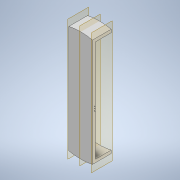
# Autodesk Inventor part: capFor6inchSch40Pipe
Saved by Autodesk Inventor 2021.1 (Build 251245000, 245)
## iProperties
Created: 2020-09-22
Part Number: capFor6inchSch40Pipe
Material: Generic
Document SubType Name: Modeling
Designer: robst
Density: 1 g/cm^3
Appearance: Default
Author: robst
Autodesk Inventor part; units mm, degrees
ref_plane "XZ Plane" through (0, 0, 0) normal (0, 1, 0) x (-1, 0, 0)
ref_plane "XY Plane" through (0, 0, 0) normal (0, 0, 1) x (1, 0, 0)
sketch "Sketch1" plane through (0, 0, 0) normal (0, 0, 1) x (1, 0, 0)
  circle A0 centre (0, 0) radius 84.1375
  circle A1 centre (0, 0) radius 88.9
  dimension "d0" = 168.275
  dimension "d1" = 4.7625
  constraints: 2 centre point, 2 coincident
  measures "d0" diameter of A0
  measures "d1" radial gap between concentric circles of A1 A0
extrude "Extrusion1" add sketch "Sketch1" along normal blind 4.7625 contours A0 | A1
extrude "Extrusion2" add sketch "Sketch1" against normal blind 25.4
sketch "Sketch2" plane through (0, 0, 0) normal (0, 0, -1) x (-1, 0, 0)
  line L0 (-83.5959, 0) -> (84.1375, 0) construction
  circle A0 centre (0, 0) radius 84.1375 construction
  spline S0 degree 2 poles (-77.1102, 1.1002) (-78.0365, 1.1002) (-79.6034, 1.7254) (-80.1746, 2.3506) knots 0 0 0 1 2 2 2
  spline S1 degree 2 poles (-80.1746, 2.3506) (-80.7458, 2.9681) (-81.371, 4.8206) (-81.371, 6.0248) knots 0 0 0 1 2 2 2
  spline S2 degree 2 poles (-81.371, 6.0248) (-81.371, 7.2212) (-80.7612, 8.9965) (-80.1823, 9.6526) knots 0 0 0 1 2 2 2
  spline S3 degree 2 poles (-80.1823, 9.6526) (-79.6111, 10.2933) (-78.0519, 10.9648) (-77.087, 10.9648) knots 0 0 0 1 2 2 2
  spline S4 degree 2 poles (-77.087, 10.9648) (-76.6085, 10.9648) (-75.7671, 10.8259) (-75.4121, 10.7178) knots 0 0 0 1 2 2 2
  spline S5 degree 2 poles (-75.4121, 10.7178) (-75.1033, 10.6175) (-74.4626, 10.3319) (-74.1462, 10.1621) knots 0 0 0 1 2 2 2
  line L1 (-74.1462, 10.1621) -> (-74.1462, 8.6337)
  line L2 (-74.1462, 8.6337) -> (-74.2465, 8.6337)
  spline S6 degree 2 poles (-74.2465, 8.6337) (-74.4163, 8.7881) (-74.9412, 9.2204) (-75.3194, 9.4288) knots 0 0 0 1 2 2 2
  spline S7 degree 2 poles (-75.3194, 9.4288) (-75.6822, 9.6295) (-76.539, 9.8842) (-77.0948, 9.8842) knots 0 0 0 1 2 2 2
  spline S8 degree 2 poles (-77.0948, 9.8842) (-77.7045, 9.8842) (-78.7929, 9.3825) (-79.202, 8.9039) knots 0 0 0 1 2 2 2
  spline S9 degree 2 poles (-79.202, 8.9039) (-79.6034, 8.4176) (-80.0511, 6.9433) (-80.0511, 6.0248) knots 0 0 0 1 2 2 2
  spline S10 degree 2 poles (-80.0511, 6.0248) (-80.0511, 5.0445) (-79.5802, 3.632) (-79.1711, 3.1457) knots 0 0 0 1 2 2 2
  spline S11 degree 2 poles (-79.1711, 3.1457) (-78.7697, 2.6748) (-77.6968, 2.1963) (-77.0948, 2.1963) knots 0 0 0 1 2 2 2
  spline S12 degree 2 poles (-77.0948, 2.1963) (-76.5467, 2.1963) (-75.6127, 2.4664) (-75.25, 2.6671) knots 0 0 0 1 2 2 2
  spline S13 degree 2 poles (-75.25, 2.6671) (-74.9026, 2.8678) (-74.3855, 3.2846) (-74.2388, 3.4313) knots 0 0 0 1 2 2 2
  line L3 (-74.2388, 3.4313) -> (-74.1462, 3.4313)
  line L4 (-74.1462, 3.4313) -> (-74.1462, 1.9184)
  spline S14 degree 2 poles (-74.1462, 1.9184) (-74.4626, 1.7717) (-75.0184, 1.5016) (-75.4121, 1.3781) knots 0 0 0 1 2 2 2
  spline S15 degree 2 poles (-75.4121, 1.3781) (-75.8289, 1.2391) (-76.539, 1.1002) (-77.1102, 1.1002) knots 0 0 0 1 2 2 2
  spline S16 degree 2 poles (-69.0749, 2.0264) (-69.2216, 1.9184) (-69.7156, 1.5324) (-69.9471, 1.4167) knots 0 0 0 1 2 2 2
  spline S17 degree 2 poles (-69.9471, 1.4167) (-70.2636, 1.2468) (-70.858, 1.0693) (-71.3983, 1.0693) knots 0 0 0 1 2 2 2
  spline S18 degree 2 poles (-71.3983, 1.0693) (-71.8383, 1.0693) (-72.6333, 1.4012) (-72.9343, 1.7023) knots 0 0 0 1 2 2 2
  spline S19 degree 2 poles (-72.9343, 1.7023) (-73.2199, 1.9956) (-73.5673, 2.8601) (-73.5673, 3.3386) knots 0 0 0 1 2 2 2
  spline S20 degree 2 poles (-73.5673, 3.3386) (-73.5673, 4.0796) (-72.942, 5.1294) (-72.2628, 5.4304) knots 0 0 0 1 2 2 2
  spline S21 degree 2 poles (-72.2628, 5.4304) (-71.6607, 5.7083) (-70.0243, 5.9167) (-69.0749, 5.9707) knots 0 0 0 1 2 2 2
  line L5 (-69.0749, 5.9707) -> (-69.0749, 6.2023)
  spline S22 degree 2 poles (-69.0749, 6.2023) (-69.0749, 6.6191) (-69.3296, 7.1363) (-69.5612, 7.2829) knots 0 0 0 1 2 2 2
  spline S23 degree 2 poles (-69.5612, 7.2829) (-69.7928, 7.4296) (-70.4566, 7.5222) (-70.8117, 7.5222) knots 0 0 0 1 2 2 2
  spline S24 degree 2 poles (-70.8117, 7.5222) (-71.2285, 7.5222) (-72.3554, 7.2752) (-72.9189, 7.0359) knots 0 0 0 1 2 2 2
  line L6 (-72.9189, 7.0359) -> (-72.9884, 7.0359)
  line L7 (-72.9884, 7.0359) -> (-72.9884, 8.2632)
  spline S25 degree 2 poles (-72.9884, 8.2632) (-72.6564, 8.3559) (-71.4137, 8.5874) (-70.8039, 8.5874) knots 0 0 0 1 2 2 2
  spline S26 degree 2 poles (-70.8039, 8.5874) (-70.0629, 8.5874) (-69.0518, 8.3559) (-68.6504, 8.0548) knots 0 0 0 1 2 2 2
  spline S27 degree 2 poles (-68.6504, 8.0548) (-68.2567, 7.7615) (-67.8708, 6.8275) (-67.8708, 6.156) knots 0 0 0 1 2 2 2
  line L8 (-67.8708, 6.156) -> (-67.8708, 1.27)
  line L9 (-67.8708, 1.27) -> (-69.0749, 1.27)
  line L10 (-69.0749, 1.27) -> (-69.0749, 2.0264)
  line L11 (-69.0749, 3.0299) -> (-69.0749, 5.0136)
  spline S28 degree 2 poles (-69.0749, 5.0136) (-69.5072, 4.975) (-70.8117, 4.8438) (-71.2208, 4.7203) knots 0 0 0 1 2 2 2
  spline S29 degree 2 poles (-71.2208, 4.7203) (-71.6993, 4.5736) (-72.3245, 3.9639) (-72.3245, 3.4235) knots 0 0 0 1 2 2 2
  spline S30 degree 2 poles (-72.3245, 3.4235) (-72.3245, 2.806) (-71.6298, 2.1808) (-70.966, 2.1808) knots 0 0 0 1 2 2 2
  spline S31 degree 2 poles (-70.966, 2.1808) (-70.4026, 2.1808) (-69.4763, 2.6671) (-69.0749, 3.0299) knots 0 0 0 1 2 2 2
  spline S32 degree 2 poles (-60.1906, 5.0368) (-60.1906, 3.246) (-61.8964, 1.1311) (-63.2009, 1.1311) knots 0 0 0 1 2 2 2
  spline S33 degree 2 poles (-63.2009, 1.1311) (-63.7335, 1.1311) (-64.5517, 1.3781) (-64.9762, 1.6328) knots 0 0 0 1 2 2 2
  line L12 (-64.9762, 1.6328) -> (-64.9762, -1.3621)
  line L13 (-64.9762, -1.3621) -> (-66.1804, -1.3621)
  line L14 (-66.1804, -1.3621) -> (-66.1804, 8.4176)
  line L15 (-66.1804, 8.4176) -> (-64.9762, 8.4176)
  line L16 (-64.9762, 8.4176) -> (-64.9762, 7.6689)
  spline S34 degree 2 poles (-64.9762, 7.6689) (-64.5286, 8.078) (-63.4325, 8.6183) (-62.7918, 8.6183) knots 0 0 0 1 2 2 2
  spline S35 degree 2 poles (-62.7918, 8.6183) (-61.5645, 8.6183) (-60.1906, 6.6732) (-60.1906, 5.0368) knots 0 0 0 1 2 2 2
  spline S36 degree 2 poles (-61.4333, 4.8978) (-61.4333, 6.1251) (-62.2129, 7.4759) (-63.0851, 7.4759) knots 0 0 0 1 2 2 2
  spline S37 degree 2 poles (-63.0851, 7.4759) (-63.5946, 7.4759) (-64.5517, 7.0205) (-64.9762, 6.6654) knots 0 0 0 1 2 2 2
  line L17 (-64.9762, 6.6654) -> (-64.9762, 2.6054)
  spline S38 degree 2 poles (-64.9762, 2.6054) (-64.5054, 2.3815) (-63.8339, 2.2117) (-63.4016, 2.2117) knots 0 0 0 1 2 2 2
  spline S39 degree 2 poles (-63.4016, 2.2117) (-62.4676, 2.2117) (-61.4333, 3.5856) (-61.4333, 4.8978) knots 0 0 0 1 2 2 2
  line L18 (-49.0601, 9.6681) -> (-53.4907, 9.6681)
  line L19 (-53.4907, 9.6681) -> (-53.4907, 6.9819)
  line L20 (-53.4907, 6.9819) -> (-49.2453, 6.9819)
  line L21 (-49.2453, 6.9819) -> (-49.2453, 5.855)
  line L22 (-49.2453, 5.855) -> (-53.4907, 5.855)
  line L23 (-53.4907, 5.855) -> (-53.4907, 1.27)
  line L24 (-53.4907, 1.27) -> (-54.7566, 1.27)
  line L25 (-54.7566, 1.27) -> (-54.7566, 10.795)
  line L26 (-54.7566, 10.795) -> (-49.0601, 10.795)
  line L27 (-49.0601, 10.795) -> (-49.0601, 9.6681)
  spline S40 degree 2 poles (-42.144, 4.8438) (-42.144, 3.0376) (-43.8808, 1.0693) (-45.3319, 1.0693) knots 0 0 0 1 2 2 2
  spline S41 degree 2 poles (-45.3319, 1.0693) (-46.8216, 1.0693) (-48.5275, 3.0994) (-48.5275, 4.8438) knots 0 0 0 1 2 2 2
  spline S42 degree 2 poles (-48.5275, 4.8438) (-48.5275, 6.6346) (-46.7676, 8.6183) (-45.3319, 8.6183) knots 0 0 0 1 2 2 2
  spline S43 degree 2 poles (-45.3319, 8.6183) (-43.8808, 8.6183) (-42.144, 6.6423) (-42.144, 4.8438) knots 0 0 0 1 2 2 2
  spline S44 degree 2 poles (-43.3868, 4.8438) (-43.3868, 6.2332) (-44.3979, 7.584) (-45.3319, 7.584) knots 0 0 0 1 2 2 2
  spline S45 degree 2 poles (-45.3319, 7.584) (-46.2659, 7.584) (-47.2848, 6.2332) (-47.2848, 4.8438) knots 0 0 0 1 2 2 2
  spline S46 degree 2 poles (-47.2848, 4.8438) (-47.2848, 3.493) (-46.2659, 2.1036) (-45.3319, 2.1036) knots 0 0 0 1 2 2 2
  spline S47 degree 2 poles (-45.3319, 2.1036) (-44.4056, 2.1036) (-43.3868, 3.4699) (-43.3868, 4.8438) knots 0 0 0 1 2 2 2
  line L28 (-37.1191, 7.1286) -> (-37.1808, 7.1286)
  spline S48 degree 2 poles (-37.1808, 7.1286) (-37.3198, 7.1672) (-37.6208, 7.1826) (-37.8292, 7.1826) knots 0 0 0 1 2 2 2
  spline S49 degree 2 poles (-37.8292, 7.1826) (-38.3155, 7.1826) (-39.2726, 6.7581) (-39.7049, 6.3413) knots 0 0 0 1 2 2 2
  line L29 (-39.7049, 6.3413) -> (-39.7049, 1.27)
  line L30 (-39.7049, 1.27) -> (-40.909, 1.27)
  line L31 (-40.909, 1.27) -> (-40.909, 8.4176)
  line L32 (-40.909, 8.4176) -> (-39.7049, 8.4176)
  line L33 (-39.7049, 8.4176) -> (-39.7049, 7.3524)
  spline S50 degree 2 poles (-39.7049, 7.3524) (-39.0488, 7.939) (-38.0685, 8.4176) (-37.6054, 8.4176) knots 0 0 0 1 2 2 2
  spline S51 degree 2 poles (-37.6054, 8.4176) (-37.4201, 8.4176) (-37.2349, 8.4022) (-37.1191, 8.379) knots 0 0 0 1 2 2 2
  line L34 (-37.1191, 8.379) -> (-37.1191, 7.1286)
  spline S52 degree 2 poles (-26.251, 4.3575) (-26.251, 3.6242) (-26.7373, 2.3815) (-27.1464, 1.9647) knots 0 0 0 1 2 2 2
  spline S53 degree 2 poles (-27.1464, 1.9647) (-27.5709, 1.5247) (-28.6361, 1.0693) (-29.2768, 1.0693) knots 0 0 0 1 2 2 2
  spline S54 degree 2 poles (-29.2768, 1.0693) (-29.9175, 1.0693) (-30.9749, 1.5016) (-31.3763, 1.9338) knots 0 0 0 1 2 2 2
  spline S55 degree 2 poles (-31.3763, 1.9338) (-31.8703, 2.451) (-32.4261, 4.1877) (-32.4261, 5.4536) knots 0 0 0 1 2 2 2
  spline S56 degree 2 poles (-32.4261, 5.4536) (-32.4261, 6.6963) (-31.9166, 8.6955) (-31.384, 9.4365) knots 0 0 0 1 2 2 2
  spline S57 degree 2 poles (-31.384, 9.4365) (-30.8669, 10.1621) (-29.2305, 10.9725) (-28.1576, 10.9725) knots 0 0 0 1 2 2 2
  spline S58 degree 2 poles (-28.1576, 10.9725) (-27.8411, 10.9725) (-27.2853, 10.9108) (-27.0769, 10.8413) knots 0 0 0 1 2 2 2
  line L35 (-27.0769, 10.8413) -> (-27.0769, 9.614)
  line L36 (-27.0769, 9.614) -> (-27.131, 9.614)
  spline S59 degree 2 poles (-27.131, 9.614) (-27.3085, 9.7066) (-27.9569, 9.8687) (-28.3274, 9.8687) knots 0 0 0 1 2 2 2
  spline S60 degree 2 poles (-28.3274, 9.8687) (-29.5161, 9.8687) (-30.9749, 8.2632) (-31.1139, 6.6886) knots 0 0 0 1 2 2 2
  spline S61 degree 2 poles (-31.1139, 6.6886) (-30.6585, 7.0051) (-29.7013, 7.3524) (-29.1301, 7.3524) knots 0 0 0 1 2 2 2
  spline S62 degree 2 poles (-29.1301, 7.3524) (-28.5744, 7.3524) (-27.7407, 7.1286) (-27.2853, 6.7889) knots 0 0 0 1 2 2 2
  spline S63 degree 2 poles (-27.2853, 6.7889) (-26.7605, 6.3953) (-26.251, 5.1757) (-26.251, 4.3575) knots 0 0 0 1 2 2 2
  spline S64 degree 2 poles (-27.5478, 4.3035) (-27.5478, 4.8901) (-27.8565, 5.6852) (-28.1962, 5.963) knots 0 0 0 1 2 2 2
  spline S65 degree 2 poles (-28.1962, 5.963) (-28.4509, 6.1637) (-29.0838, 6.2949) (-29.4157, 6.2949) knots 0 0 0 1 2 2 2
  spline S66 degree 2 poles (-29.4157, 6.2949) (-29.8634, 6.2949) (-30.7048, 6.0248) (-31.1139, 5.7701) knots 0 0 0 1 2 2 2
  spline S67 degree 2 poles (-31.1139, 5.7701) (-31.1216, 5.6311) (-31.137, 5.3687) (-31.137, 5.168) knots 0 0 0 1 2 2 2
  spline S68 degree 2 poles (-31.137, 5.168) (-31.137, 4.18) (-30.7511, 2.9681) (-30.4578, 2.6517) knots 0 0 0 1 2 2 2
  spline S69 degree 2 poles (-30.4578, 2.6517) (-30.1876, 2.3506) (-29.601, 2.1113) (-29.2691, 2.1113) knots 0 0 0 1 2 2 2
  spline S70 degree 2 poles (-29.2691, 2.1113) (-28.4972, 2.1113) (-27.5478, 3.2074) (-27.5478, 4.3035) knots 0 0 0 1 2 2 2
  line L37 (-21.2878, 11.2195) -> (-21.5657, 7.5145)
  line L38 (-21.5657, 7.5145) -> (-22.4071, 7.5145)
  line L39 (-22.4071, 7.5145) -> (-22.6849, 11.2195)
  line L40 (-22.6849, 11.2195) -> (-21.2878, 11.2195)
  line L41 (-23.6961, 11.2195) -> (-23.974, 7.5145)
  line L42 (-23.974, 7.5145) -> (-24.8153, 7.5145)
  line L43 (-24.8153, 7.5145) -> (-25.0932, 11.2195)
  line L44 (-25.0932, 11.2195) -> (-23.6961, 11.2195)
  spline S71 degree 2 poles (-12.8512, 1.1002) (-13.8855, 1.1002) (-15.3366, 1.5324) (-15.9773, 1.8412) knots 0 0 0 1 2 2 2
  line L45 (-15.9773, 1.8412) -> (-15.9773, 3.4313)
  line L46 (-15.9773, 3.4313) -> (-15.8847, 3.4313)
  spline S72 degree 2 poles (-15.8847, 3.4313) (-15.2594, 2.8446) (-13.6771, 2.1963) (-12.9438, 2.1963) knots 0 0 0 1 2 2 2
  spline S73 degree 2 poles (-12.9438, 2.1963) (-11.8941, 2.1963) (-10.8211, 3.0685) (-10.8211, 3.7863) knots 0 0 0 1 2 2 2
  spline S74 degree 2 poles (-10.8211, 3.7863) (-10.8211, 4.3575) (-11.3846, 5.0676) (-11.9944, 5.2452) knots 0 0 0 1 2 2 2
  spline S75 degree 2 poles (-11.9944, 5.2452) (-12.4344, 5.3687) (-13.1677, 5.5385) (-13.7157, 5.6774) knots 0 0 0 1 2 2 2
  spline S76 degree 2 poles (-13.7157, 5.6774) (-14.2097, 5.8087) (-14.9893, 6.2023) (-15.2903, 6.5188) knots 0 0 0 1 2 2 2
  spline S77 degree 2 poles (-15.2903, 6.5188) (-15.5836, 6.8353) (-15.9078, 7.6843) (-15.9078, 8.2401) knots 0 0 0 1 2 2 2
  spline S78 degree 2 poles (-15.9078, 8.2401) (-15.9078, 9.3979) (-14.1016, 10.9648) (-12.7045, 10.9648) knots 0 0 0 1 2 2 2
  spline S79 degree 2 poles (-12.7045, 10.9648) (-11.9018, 10.9648) (-10.4815, 10.6483) (-9.8717, 10.3473) knots 0 0 0 1 2 2 2
  line L47 (-9.8717, 10.3473) -> (-9.8717, 8.8344)
  line L48 (-9.8717, 8.8344) -> (-9.9644, 8.8344)
  spline S80 degree 2 poles (-9.9644, 8.8344) (-10.4198, 9.2512) (-11.84, 9.8687) (-12.6196, 9.8687) knots 0 0 0 1 2 2 2
  spline S81 degree 2 poles (-12.6196, 9.8687) (-13.4996, 9.8687) (-14.5879, 9.0428) (-14.5879, 8.3713) knots 0 0 0 1 2 2 2
  spline S82 degree 2 poles (-14.5879, 8.3713) (-14.5879, 7.7692) (-13.9473, 7.0514) (-13.3452, 6.8893) knots 0 0 0 1 2 2 2
  spline S83 degree 2 poles (-13.3452, 6.8893) (-12.9438, 6.7812) (-11.7783, 6.5033) (-11.3923, 6.3876) knots 0 0 0 1 2 2 2
  spline S84 degree 2 poles (-11.3923, 6.3876) (-10.412, 6.0865) (-9.5012, 4.8747) (-9.5012, 3.987) knots 0 0 0 1 2 2 2
  spline S85 degree 2 poles (-9.5012, 3.987) (-9.5012, 3.4235) (-9.9566, 2.3429) (-10.3657, 1.9647) knots 0 0 0 1 2 2 2
  spline S86 degree 2 poles (-10.3657, 1.9647) (-10.8211, 1.5479) (-11.979, 1.1002) (-12.8512, 1.1002) knots 0 0 0 1 2 2 2
  spline S87 degree 2 poles (-5.4643, 1.1079) (-6.2053, 1.1079) (-7.4326, 1.5633) (-7.8726, 2.0264) knots 0 0 0 1 2 2 2
  spline S88 degree 2 poles (-7.8726, 2.0264) (-8.3125, 2.4819) (-8.7988, 3.8867) (-8.7988, 4.8284) knots 0 0 0 1 2 2 2
  spline S89 degree 2 poles (-8.7988, 4.8284) (-8.7988, 5.7701) (-8.2971, 7.144) (-7.8726, 7.6071) knots 0 0 0 1 2 2 2
  spline S90 degree 2 poles (-7.8726, 7.6071) (-7.448, 8.078) (-6.1899, 8.5797) (-5.4643, 8.5797) knots 0 0 0 1 2 2 2
  spline S91 degree 2 poles (-5.4643, 8.5797) (-4.8777, 8.5797) (-3.7816, 8.2478) (-3.3571, 8.0317) knots 0 0 0 1 2 2 2
  line L49 (-3.3571, 8.0317) -> (-3.3571, 6.6809)
  line L50 (-3.3571, 6.6809) -> (-3.4265, 6.6809)
  spline S92 degree 2 poles (-3.4265, 6.6809) (-3.5577, 6.7889) (-3.9591, 7.0668) (-4.2447, 7.2135) knots 0 0 0 1 2 2 2
  spline S93 degree 2 poles (-4.2447, 7.2135) (-4.4994, 7.337) (-5.1787, 7.5299) (-5.4874, 7.5299) knots 0 0 0 1 2 2 2
  spline S94 degree 2 poles (-5.4874, 7.5299) (-6.4214, 7.5299) (-7.5561, 6.1174) (-7.5561, 4.8284) knots 0 0 0 1 2 2 2
  spline S95 degree 2 poles (-7.5561, 4.8284) (-7.5561, 3.5702) (-6.46, 2.1577) (-5.4874, 2.1577) knots 0 0 0 1 2 2 2
  spline S96 degree 2 poles (-5.4874, 2.1577) (-4.9008, 2.1577) (-3.8356, 2.6439) (-3.4265, 3.0222) knots 0 0 0 1 2 2 2
  line L51 (-3.4265, 3.0222) -> (-3.3571, 3.0222)
  line L52 (-3.3571, 3.0222) -> (-3.3571, 1.6714)
  spline S97 degree 2 poles (-3.3571, 1.6714) (-3.5346, 1.5865) (-4.0749, 1.3472) (-4.291, 1.2932) knots 0 0 0 1 2 2 2
  spline S98 degree 2 poles (-4.291, 1.2932) (-4.5998, 1.2005) (-5.0861, 1.1079) (-5.4643, 1.1079) knots 0 0 0 1 2 2 2
  line L53 (3.3506, 1.27) -> (2.1464, 1.27)
  line L54 (2.1464, 1.27) -> (2.1464, 5.3455)
  spline S99 degree 2 poles (2.1464, 5.3455) (2.1464, 5.8395) (2.0538, 6.6886) (1.9149, 6.9433) knots 0 0 0 1 2 2 2
  spline S100 degree 2 poles (1.9149, 6.9433) (1.7682, 7.2135) (1.2433, 7.4759) (0.7957, 7.4759) knots 0 0 0 1 2 2 2
  spline S101 degree 2 poles (0.7957, 7.4759) (0.348, 7.4759) (-0.6014, 6.9973) (-1.0569, 6.6114) knots 0 0 0 1 2 2 2
  line L55 (-1.0569, 6.6114) -> (-1.0569, 1.27)
  line L56 (-1.0569, 1.27) -> (-2.261, 1.27)
  line L57 (-2.261, 1.27) -> (-2.261, 11.2195)
  line L58 (-2.261, 11.2195) -> (-1.0569, 11.2195)
  line L59 (-1.0569, 11.2195) -> (-1.0569, 7.6226)
  spline S102 degree 2 poles (-1.0569, 7.6226) (-0.5165, 8.1089) (0.5255, 8.6183) (1.1121, 8.6183) knots 0 0 0 1 2 2 2
  spline S103 degree 2 poles (1.1121, 8.6183) (2.1619, 8.6183) (3.3506, 7.2289) (3.3506, 5.909) knots 0 0 0 1 2 2 2
  line L60 (3.3506, 5.909) -> (3.3506, 1.27)
  spline S104 degree 2 poles (8.144, 1.1079) (6.4304, 1.1079) (4.547, 3.0299) (4.547, 4.8052) knots 0 0 0 1 2 2 2
  spline S105 degree 2 poles (4.547, 4.8052) (4.547, 6.5497) (6.3763, 8.6183) (7.8506, 8.6183) knots 0 0 0 1 2 2 2
  spline S106 degree 2 poles (7.8506, 8.6183) (8.5145, 8.6183) (9.5411, 8.2324) (9.9193, 7.8233) knots 0 0 0 1 2 2 2
  spline S107 degree 2 poles (9.9193, 7.8233) (10.3052, 7.4142) (10.7143, 6.2332) (10.7143, 5.3764) knots 0 0 0 1 2 2 2
  line L61 (10.7143, 5.3764) -> (10.7143, 4.7203)
  line L62 (10.7143, 4.7203) -> (5.7666, 4.7203)
  spline S108 degree 2 poles (5.7666, 4.7203) (5.7666, 3.4776) (7.017, 2.1577) (8.1285, 2.1577) knots 0 0 0 1 2 2 2
  spline S109 degree 2 poles (8.1285, 2.1577) (8.5222, 2.1577) (9.2863, 2.3352) (9.5951, 2.4741) knots 0 0 0 1 2 2 2
  spline S110 degree 2 poles (9.5951, 2.4741) (9.9193, 2.6285) (10.367, 2.8987) (10.5136, 3.0222) knots 0 0 0 1 2 2 2
  line L63 (10.5136, 3.0222) -> (10.5831, 3.0222)
  line L64 (10.5831, 3.0222) -> (10.5831, 1.71)
  spline S111 degree 2 poles (10.5831, 1.71) (10.3747, 1.6251) (9.7417, 1.3781) (9.4947, 1.3086) knots 0 0 0 1 2 2 2
  spline S112 degree 2 poles (9.4947, 1.3086) (9.1474, 1.2082) (8.5762, 1.1079) (8.144, 1.1079) knots 0 0 0 1 2 2 2
  spline S113 degree 2 poles (9.5411, 5.6388) (9.5256, 6.1251) (9.3249, 6.8353) (9.132, 7.0745) knots 0 0 0 1 2 2 2
  spline S114 degree 2 poles (9.132, 7.0745) (8.9236, 7.3447) (8.2675, 7.6303) (7.7812, 7.6303) knots 0 0 0 1 2 2 2
  spline S115 degree 2 poles (7.7812, 7.6303) (7.3026, 7.6303) (6.6311, 7.3447) (6.3532, 7.0668) knots 0 0 0 1 2 2 2
  spline S116 degree 2 poles (6.3532, 7.0668) (6.083, 6.7812) (5.8052, 6.0943) (5.7666, 5.6388) knots 0 0 0 1 2 2 2
  line L65 (5.7666, 5.6388) -> (9.5411, 5.6388)
  line L66 (17.4297, 1.27) -> (16.2255, 1.27)
  line L67 (16.2255, 1.27) -> (16.2255, 1.9956)
  spline S117 degree 2 poles (16.2255, 1.9956) (15.9477, 1.764) (15.5386, 1.4553) (15.2607, 1.324) knots 0 0 0 1 2 2 2
  spline S118 degree 2 poles (15.2607, 1.324) (15.006, 1.2005) (14.4579, 1.0693) (14.0951, 1.0693) knots 0 0 0 1 2 2 2
  spline S119 degree 2 poles (14.0951, 1.0693) (13.5085, 1.0693) (12.5205, 1.5556) (12.1732, 2.0264) knots 0 0 0 1 2 2 2
  spline S120 degree 2 poles (12.1732, 2.0264) (11.8258, 2.4973) (11.4399, 3.8867) (11.4399, 4.7898) knots 0 0 0 1 2 2 2
  spline S121 degree 2 poles (11.4399, 4.7898) (11.4399, 5.7315) (11.9262, 7.1054) (12.3507, 7.6226) knots 0 0 0 1 2 2 2
  spline S122 degree 2 poles (12.3507, 7.6226) (12.7444, 8.0857) (13.8481, 8.6183) (14.4579, 8.6183) knots 0 0 0 1 2 2 2
  spline S123 degree 2 poles (14.4579, 8.6183) (14.9905, 8.6183) (15.7856, 8.379) (16.2255, 8.132) knots 0 0 0 1 2 2 2
  line L68 (16.2255, 8.132) -> (16.2255, 11.2195)
  line L69 (16.2255, 11.2195) -> (17.4297, 11.2195)
  line L70 (17.4297, 11.2195) -> (17.4297, 1.27)
  line L71 (16.2255, 3.0067) -> (16.2255, 7.1363)
  spline S124 degree 2 poles (16.2255, 7.1363) (15.7778, 7.3524) (15.0677, 7.5145) (14.6586, 7.5145) knots 0 0 0 1 2 2 2
  spline S125 degree 2 poles (14.6586, 7.5145) (13.7324, 7.5145) (12.6826, 6.1251) (12.6826, 4.8129) knots 0 0 0 1 2 2 2
  spline S126 degree 2 poles (12.6826, 4.8129) (12.6826, 3.547) (13.4854, 2.2117) (14.373, 2.2117) knots 0 0 0 1 2 2 2
  spline S127 degree 2 poles (14.373, 2.2117) (14.8439, 2.2117) (15.801, 2.6439) (16.2255, 3.0067) knots 0 0 0 1 2 2 2
  line L72 (24.7317, 1.27) -> (23.5275, 1.27)
  line L73 (23.5275, 1.27) -> (23.5275, 2.0573)
  spline S128 degree 2 poles (23.5275, 2.0573) (22.9718, 1.571) (21.976, 1.0693) (21.3585, 1.0693) knots 0 0 0 1 2 2 2
  spline S129 degree 2 poles (21.3585, 1.0693) (20.8954, 1.0693) (20.0695, 1.3781) (19.7685, 1.71) knots 0 0 0 1 2 2 2
  spline S130 degree 2 poles (19.7685, 1.71) (19.4597, 2.0419) (19.1201, 3.053) (19.1201, 3.7786) knots 0 0 0 1 2 2 2
  line L74 (19.1201, 3.7786) -> (19.1201, 8.4176)
  line L75 (19.1201, 8.4176) -> (20.3242, 8.4176)
  line L76 (20.3242, 8.4176) -> (20.3242, 4.3421)
  spline S131 degree 2 poles (20.3242, 4.3421) (20.3242, 3.7709) (20.4091, 3.0222) (20.5558, 2.7443) knots 0 0 0 1 2 2 2
  spline S132 degree 2 poles (20.5558, 2.7443) (20.7024, 2.4664) (21.2042, 2.2117) (21.675, 2.2117) knots 0 0 0 1 2 2 2
  spline S133 degree 2 poles (21.675, 2.2117) (22.115, 2.2117) (23.1107, 2.7134) (23.5275, 3.0762) knots 0 0 0 1 2 2 2
  line L77 (23.5275, 3.0762) -> (23.5275, 8.4176)
  line L78 (23.5275, 8.4176) -> (24.7317, 8.4176)
  line L79 (24.7317, 8.4176) -> (24.7317, 1.27)
  line L80 (27.7034, 1.27) -> (26.4993, 1.27)
  line L81 (26.4993, 1.27) -> (26.4993, 11.2195)
  line L82 (26.4993, 11.2195) -> (27.7034, 11.2195)
  line L83 (27.7034, 11.2195) -> (27.7034, 1.27)
  spline S134 degree 2 poles (32.574, 1.1079) (30.8604, 1.1079) (28.977, 3.0299) (28.977, 4.8052) knots 0 0 0 1 2 2 2
  spline S135 degree 2 poles (28.977, 4.8052) (28.977, 6.5497) (30.8064, 8.6183) (32.2806, 8.6183) knots 0 0 0 1 2 2 2
  spline S136 degree 2 poles (32.2806, 8.6183) (32.9445, 8.6183) (33.9711, 8.2324) (34.3493, 7.8233) knots 0 0 0 1 2 2 2
  spline S137 degree 2 poles (34.3493, 7.8233) (34.7352, 7.4142) (35.1443, 6.2332) (35.1443, 5.3764) knots 0 0 0 1 2 2 2
  line L84 (35.1443, 5.3764) -> (35.1443, 4.7203)
  line L85 (35.1443, 4.7203) -> (30.1966, 4.7203)
  spline S138 degree 2 poles (30.1966, 4.7203) (30.1966, 3.4776) (31.447, 2.1577) (32.5585, 2.1577) knots 0 0 0 1 2 2 2
  spline S139 degree 2 poles (32.5585, 2.1577) (32.9522, 2.1577) (33.7163, 2.3352) (34.0251, 2.4741) knots 0 0 0 1 2 2 2
  spline S140 degree 2 poles (34.0251, 2.4741) (34.3493, 2.6285) (34.797, 2.8987) (34.9436, 3.0222) knots 0 0 0 1 2 2 2
  line L86 (34.9436, 3.0222) -> (35.0131, 3.0222)
  line L87 (35.0131, 3.0222) -> (35.0131, 1.71)
  spline S141 degree 2 poles (35.0131, 1.71) (34.8047, 1.6251) (34.1717, 1.3781) (33.9247, 1.3086) knots 0 0 0 1 2 2 2
  spline S142 degree 2 poles (33.9247, 1.3086) (33.5774, 1.2082) (33.0062, 1.1079) (32.574, 1.1079) knots 0 0 0 1 2 2 2
  spline S143 degree 2 poles (33.9711, 5.6388) (33.9556, 6.1251) (33.7549, 6.8353) (33.562, 7.0745) knots 0 0 0 1 2 2 2
  spline S144 degree 2 poles (33.562, 7.0745) (33.3536, 7.3447) (32.6975, 7.6303) (32.2112, 7.6303) knots 0 0 0 1 2 2 2
  spline S145 degree 2 poles (32.2112, 7.6303) (31.7326, 7.6303) (31.0611, 7.3447) (30.7832, 7.0668) knots 0 0 0 1 2 2 2
  spline S146 degree 2 poles (30.7832, 7.0668) (30.513, 6.7812) (30.2352, 6.0943) (30.1966, 5.6388) knots 0 0 0 1 2 2 2
  line L88 (30.1966, 5.6388) -> (33.9711, 5.6388)
  line L89 (46.406, 4.5428) -> (45.2714, 4.5428)
  line L90 (45.2714, 4.5428) -> (45.2714, 1.27)
  line L91 (45.2714, 1.27) -> (44.0441, 1.27)
  line L92 (44.0441, 1.27) -> (44.0441, 4.5428)
  line L93 (44.0441, 4.5428) -> (39.8373, 4.5428)
  line L94 (39.8373, 4.5428) -> (39.8373, 5.8858)
  line L95 (39.8373, 5.8858) -> (44.0981, 10.795)
  line L96 (44.0981, 10.795) -> (45.2714, 10.795)
  line L97 (45.2714, 10.795) -> (45.2714, 5.5694)
  line L98 (45.2714, 5.5694) -> (46.406, 5.5694)
  line L99 (46.406, 5.5694) -> (46.406, 4.5428)
  line L100 (44.0441, 5.5694) -> (44.0441, 9.2898)
  line L101 (44.0441, 9.2898) -> (40.8408, 5.5694)
  line L102 (40.8408, 5.5694) -> (44.0441, 5.5694)
  spline S147 degree 2 poles (53.353, 6.0325) (53.353, 3.4699) (51.8632, 1.0693) (50.3118, 1.0693) knots 0 0 0 1 2 2 2
  spline S148 degree 2 poles (50.3118, 1.0693) (48.7371, 1.0693) (47.2628, 3.5162) (47.2628, 6.0248) knots 0 0 0 1 2 2 2
  spline S149 degree 2 poles (47.2628, 6.0248) (47.2628, 8.6029) (48.7526, 10.988) (50.3118, 10.988) knots 0 0 0 1 2 2 2
  spline S150 degree 2 poles (50.3118, 10.988) (51.8787, 10.988) (53.353, 8.518) (53.353, 6.0325) knots 0 0 0 1 2 2 2
  spline S151 degree 2 poles (51.7166, 3.1302) (51.9018, 3.6011) (52.0562, 5.0522) (52.0562, 6.0325) knots 0 0 0 1 2 2 2
  spline S152 degree 2 poles (52.0562, 6.0325) (52.0562, 7.0128) (51.9018, 8.4562) (51.7089, 8.9425) knots 0 0 0 1 2 2 2
  spline S153 degree 2 poles (51.7089, 8.9425) (51.5159, 9.4288) (50.8444, 9.9305) (50.3118, 9.9305) knots 0 0 0 1 2 2 2
  spline S154 degree 2 poles (50.3118, 9.9305) (49.7792, 9.9305) (49.0922, 9.4288) (48.8915, 8.9271) knots 0 0 0 1 2 2 2
  spline S155 degree 2 poles (48.8915, 8.9271) (48.6985, 8.4408) (48.5596, 6.9588) (48.5596, 6.0248) knots 0 0 0 1 2 2 2
  spline S156 degree 2 poles (48.5596, 6.0248) (48.5596, 5.0213) (48.6831, 3.6783) (48.8838, 3.1534) knots 0 0 0 1 2 2 2
  spline S157 degree 2 poles (48.8838, 3.1534) (49.069, 2.6594) (49.756, 2.1268) (50.3118, 2.1268) knots 0 0 0 1 2 2 2
  spline S158 degree 2 poles (50.3118, 2.1268) (50.8366, 2.1268) (51.5236, 2.6285) (51.7166, 3.1302) knots 0 0 0 1 2 2 2
  spline S159 degree 2 poles (64.8308, 5.0368) (64.8308, 3.246) (63.125, 1.1311) (61.8205, 1.1311) knots 0 0 0 1 2 2 2
  spline S160 degree 2 poles (61.8205, 1.1311) (61.2879, 1.1311) (60.4697, 1.3781) (60.0452, 1.6328) knots 0 0 0 1 2 2 2
  line L103 (60.0452, 1.6328) -> (60.0452, -1.3621)
  line L104 (60.0452, -1.3621) -> (58.841, -1.3621)
  line L105 (58.841, -1.3621) -> (58.841, 8.4176)
  line L106 (58.841, 8.4176) -> (60.0452, 8.4176)
  line L107 (60.0452, 8.4176) -> (60.0452, 7.6689)
  spline S161 degree 2 poles (60.0452, 7.6689) (60.4929, 8.078) (61.5889, 8.6183) (62.2296, 8.6183) knots 0 0 0 1 2 2 2
  spline S162 degree 2 poles (62.2296, 8.6183) (63.4569, 8.6183) (64.8308, 6.6732) (64.8308, 5.0368) knots 0 0 0 1 2 2 2
  spline S163 degree 2 poles (63.5881, 4.8978) (63.5881, 6.1251) (62.8085, 7.4759) (61.9363, 7.4759) knots 0 0 0 1 2 2 2
  spline S164 degree 2 poles (61.9363, 7.4759) (61.4268, 7.4759) (60.4697, 7.0205) (60.0452, 6.6654) knots 0 0 0 1 2 2 2
  line L108 (60.0452, 6.6654) -> (60.0452, 2.6054)
  spline S165 degree 2 poles (60.0452, 2.6054) (60.516, 2.3815) (61.1875, 2.2117) (61.6198, 2.2117) knots 0 0 0 1 2 2 2
  spline S166 degree 2 poles (61.6198, 2.2117) (62.5538, 2.2117) (63.5881, 3.5856) (63.5881, 4.8978) knots 0 0 0 1 2 2 2
  line L109 (67.3086, 1.27) -> (66.1044, 1.27)
  line L110 (66.1044, 1.27) -> (66.1044, 8.4176)
  line L111 (66.1044, 8.4176) -> (67.3086, 8.4176)
  line L112 (67.3086, 8.4176) -> (67.3086, 1.27)
  line L113 (67.3935, 9.6063) -> (66.0272, 9.6063)
  line L114 (66.0272, 9.6063) -> (66.0272, 10.8568)
  line L115 (66.0272, 10.8568) -> (67.3935, 10.8568)
  line L116 (67.3935, 10.8568) -> (67.3935, 9.6063)
  spline S167 degree 2 poles (75.066, 5.0368) (75.066, 3.246) (73.3601, 1.1311) (72.0556, 1.1311) knots 0 0 0 1 2 2 2
  spline S168 degree 2 poles (72.0556, 1.1311) (71.523, 1.1311) (70.7048, 1.3781) (70.2803, 1.6328) knots 0 0 0 1 2 2 2
  line L117 (70.2803, 1.6328) -> (70.2803, -1.3621)
  line L118 (70.2803, -1.3621) -> (69.0762, -1.3621)
  line L119 (69.0762, -1.3621) -> (69.0762, 8.4176)
  line L120 (69.0762, 8.4176) -> (70.2803, 8.4176)
  line L121 (70.2803, 8.4176) -> (70.2803, 7.6689)
  spline S169 degree 2 poles (70.2803, 7.6689) (70.728, 8.078) (71.8241, 8.6183) (72.4647, 8.6183) knots 0 0 0 1 2 2 2
  spline S170 degree 2 poles (72.4647, 8.6183) (73.692, 8.6183) (75.066, 6.6732) (75.066, 5.0368) knots 0 0 0 1 2 2 2
  spline S171 degree 2 poles (73.8232, 4.8978) (73.8232, 6.1251) (73.0436, 7.4759) (72.1714, 7.4759) knots 0 0 0 1 2 2 2
  spline S172 degree 2 poles (72.1714, 7.4759) (71.662, 7.4759) (70.7048, 7.0205) (70.2803, 6.6654) knots 0 0 0 1 2 2 2
  line L122 (70.2803, 6.6654) -> (70.2803, 2.6054)
  spline S173 degree 2 poles (70.2803, 2.6054) (70.7511, 2.3815) (71.4227, 2.2117) (71.8549, 2.2117) knots 0 0 0 1 2 2 2
  spline S174 degree 2 poles (71.8549, 2.2117) (72.7889, 2.2117) (73.8232, 3.5856) (73.8232, 4.8978) knots 0 0 0 1 2 2 2
  spline S175 degree 2 poles (79.4194, 1.1079) (77.7058, 1.1079) (75.8224, 3.0299) (75.8224, 4.8052) knots 0 0 0 1 2 2 2
  spline S176 degree 2 poles (75.8224, 4.8052) (75.8224, 6.5497) (77.6517, 8.6183) (79.126, 8.6183) knots 0 0 0 1 2 2 2
  spline S177 degree 2 poles (79.126, 8.6183) (79.7899, 8.6183) (80.8165, 8.2324) (81.1947, 7.8233) knots 0 0 0 1 2 2 2
  spline S178 degree 2 poles (81.1947, 7.8233) (81.5806, 7.4142) (81.9897, 6.2332) (81.9897, 5.3764) knots 0 0 0 1 2 2 2
  line L123 (81.9897, 5.3764) -> (81.9897, 4.7203)
  line L124 (81.9897, 4.7203) -> (77.042, 4.7203)
  spline S179 degree 2 poles (77.042, 4.7203) (77.042, 3.4776) (78.2924, 2.1577) (79.4039, 2.1577) knots 0 0 0 1 2 2 2
  spline S180 degree 2 poles (79.4039, 2.1577) (79.7976, 2.1577) (80.5617, 2.3352) (80.8705, 2.4741) knots 0 0 0 1 2 2 2
  spline S181 degree 2 poles (80.8705, 2.4741) (81.1947, 2.6285) (81.6424, 2.8987) (81.789, 3.0222) knots 0 0 0 1 2 2 2
  line L125 (81.789, 3.0222) -> (81.8585, 3.0222)
  line L126 (81.8585, 3.0222) -> (81.8585, 1.71)
  spline S182 degree 2 poles (81.8585, 1.71) (81.6501, 1.6251) (81.0171, 1.3781) (80.7701, 1.3086) knots 0 0 0 1 2 2 2
  spline S183 degree 2 poles (80.7701, 1.3086) (80.4228, 1.2082) (79.8516, 1.1079) (79.4194, 1.1079) knots 0 0 0 1 2 2 2
  spline S184 degree 2 poles (80.8165, 5.6388) (80.801, 6.1251) (80.6003, 6.8353) (80.4074, 7.0745) knots 0 0 0 1 2 2 2
  spline S185 degree 2 poles (80.4074, 7.0745) (80.199, 7.3447) (79.5429, 7.6303) (79.0566, 7.6303) knots 0 0 0 1 2 2 2
  spline S186 degree 2 poles (79.0566, 7.6303) (78.578, 7.6303) (77.9065, 7.3447) (77.6286, 7.0668) knots 0 0 0 1 2 2 2
  spline S187 degree 2 poles (77.6286, 7.0668) (77.3584, 6.7812) (77.0806, 6.0943) (77.042, 5.6388) knots 0 0 0 1 2 2 2
  line L127 (77.042, 5.6388) -> (80.8165, 5.6388)
  line L128 (-22.3916, -4.9265) -> (-25.6721, -14.4515)
  line L129 (-25.6721, -14.4515) -> (-27.0383, -14.4515)
  line L130 (-27.0383, -14.4515) -> (-30.3188, -4.9265)
  line L131 (-30.3188, -4.9265) -> (-28.9603, -4.9265)
  line L132 (-28.9603, -4.9265) -> (-26.3205, -12.8382)
  line L133 (-26.3205, -12.8382) -> (-23.6807, -4.9265)
  line L134 (-23.6807, -4.9265) -> (-22.3916, -4.9265)
  spline S188 degree 2 poles (-18.3624, -14.6136) (-20.076, -14.6136) (-21.9594, -12.6916) (-21.9594, -10.9163) knots 0 0 0 1 2 2 2
  spline S189 degree 2 poles (-21.9594, -10.9163) (-21.9594, -9.1718) (-20.13, -7.1032) (-18.6557, -7.1032) knots 0 0 0 1 2 2 2
  spline S190 degree 2 poles (-18.6557, -7.1032) (-17.9919, -7.1032) (-16.9653, -7.4891) (-16.5871, -7.8982) knots 0 0 0 1 2 2 2
  spline S191 degree 2 poles (-16.5871, -7.8982) (-16.2011, -8.3073) (-15.792, -9.4883) (-15.792, -10.3451) knots 0 0 0 1 2 2 2
  line L135 (-15.792, -10.3451) -> (-15.792, -11.0012)
  line L136 (-15.792, -11.0012) -> (-20.7398, -11.0012)
  spline S192 degree 2 poles (-20.7398, -11.0012) (-20.7398, -12.2439) (-19.4893, -13.5638) (-18.3778, -13.5638) knots 0 0 0 1 2 2 2
  spline S193 degree 2 poles (-18.3778, -13.5638) (-17.9842, -13.5638) (-17.22, -13.3863) (-16.9113, -13.2473) knots 0 0 0 1 2 2 2
  spline S194 degree 2 poles (-16.9113, -13.2473) (-16.5871, -13.093) (-16.1394, -12.8228) (-15.9927, -12.6993) knots 0 0 0 1 2 2 2
  line L137 (-15.9927, -12.6993) -> (-15.9233, -12.6993)
  line L138 (-15.9233, -12.6993) -> (-15.9233, -14.0115)
  spline S195 degree 2 poles (-15.9233, -14.0115) (-16.1317, -14.0964) (-16.7646, -14.3434) (-17.0116, -14.4129) knots 0 0 0 1 2 2 2
  spline S196 degree 2 poles (-17.0116, -14.4129) (-17.359, -14.5132) (-17.9302, -14.6136) (-18.3624, -14.6136) knots 0 0 0 1 2 2 2
  spline S197 degree 2 poles (-16.9653, -10.0826) (-16.9807, -9.5964) (-17.1814, -8.8862) (-17.3744, -8.6469) knots 0 0 0 1 2 2 2
  spline S198 degree 2 poles (-17.3744, -8.6469) (-17.5828, -8.3768) (-18.2389, -8.0912) (-18.7252, -8.0912) knots 0 0 0 1 2 2 2
  spline S199 degree 2 poles (-18.7252, -8.0912) (-19.2038, -8.0912) (-19.8753, -8.3768) (-20.1532, -8.6547) knots 0 0 0 1 2 2 2
  spline S200 degree 2 poles (-20.1532, -8.6547) (-20.4233, -8.9403) (-20.7012, -9.6272) (-20.7398, -10.0826) knots 0 0 0 1 2 2 2
  line L139 (-20.7398, -10.0826) -> (-16.9653, -10.0826)
  line L140 (-10.7825, -8.5929) -> (-10.8443, -8.5929)
  spline S201 degree 2 poles (-10.8443, -8.5929) (-10.9832, -8.5543) (-11.2843, -8.5389) (-11.4927, -8.5389) knots 0 0 0 1 2 2 2
  spline S202 degree 2 poles (-11.4927, -8.5389) (-11.979, -8.5389) (-12.9361, -8.9634) (-13.3683, -9.3802) knots 0 0 0 1 2 2 2
  line L141 (-13.3683, -9.3802) -> (-13.3683, -14.4515)
  line L142 (-13.3683, -14.4515) -> (-14.5725, -14.4515)
  line L143 (-14.5725, -14.4515) -> (-14.5725, -7.3039)
  line L144 (-14.5725, -7.3039) -> (-13.3683, -7.3039)
  line L145 (-13.3683, -7.3039) -> (-13.3683, -8.3691)
  spline S203 degree 2 poles (-13.3683, -8.3691) (-12.7122, -7.7824) (-11.732, -7.3039) (-11.2688, -7.3039) knots 0 0 0 1 2 2 2
  spline S204 degree 2 poles (-11.2688, -7.3039) (-11.0836, -7.3039) (-10.8983, -7.3193) (-10.7825, -7.3425) knots 0 0 0 1 2 2 2
  line L146 (-10.7825, -7.3425) -> (-10.7825, -8.5929)
  spline S205 degree 2 poles (-7.9189, -14.6213) (-8.6367, -14.6213) (-9.8794, -14.2354) (-10.2885, -14.0192) knots 0 0 0 1 2 2 2
  line L147 (-10.2885, -14.0192) -> (-10.2885, -12.6684)
  line L148 (-10.2885, -12.6684) -> (-10.2268, -12.6684)
  spline S206 degree 2 poles (-10.2268, -12.6684) (-10.0724, -12.7919) (-9.6556, -13.0852) (-9.3083, -13.2473) knots 0 0 0 1 2 2 2
  spline S207 degree 2 poles (-9.3083, -13.2473) (-9.0072, -13.394) (-8.2662, -13.6101) (-7.8726, -13.6101) knots 0 0 0 1 2 2 2
  spline S208 degree 2 poles (-7.8726, -13.6101) (-7.587, -13.6101) (-6.9309, -13.4789) (-6.7765, -13.3708) knots 0 0 0 1 2 2 2
  spline S209 degree 2 poles (-6.7765, -13.3708) (-6.5526, -13.2242) (-6.352, -12.8923) (-6.352, -12.5527) knots 0 0 0 1 2 2 2
  spline S210 degree 2 poles (-6.352, -12.5527) (-6.352, -12.1281) (-6.8151, -11.6881) (-7.4094, -11.5415) knots 0 0 0 1 2 2 2
  spline S211 degree 2 poles (-7.4094, -11.5415) (-7.641, -11.4875) (-8.382, -11.3331) (-8.6985, -11.2482) knots 0 0 0 1 2 2 2
  spline S212 degree 2 poles (-8.6985, -11.2482) (-9.5167, -11.0089) (-10.2577, -10.0209) (-10.2577, -9.3185) knots 0 0 0 1 2 2 2
  spline S213 degree 2 poles (-10.2577, -9.3185) (-10.2577, -8.3459) (-8.7988, -7.1341) (-7.5947, -7.1341) knots 0 0 0 1 2 2 2
  spline S214 degree 2 poles (-7.5947, -7.1341) (-7.0003, -7.1341) (-5.7962, -7.4274) (-5.3871, -7.6512) knots 0 0 0 1 2 2 2
  line L149 (-5.3871, -7.6512) -> (-5.3871, -8.9403)
  line L150 (-5.3871, -8.9403) -> (-5.4489, -8.9403)
  spline S215 degree 2 poles (-5.4489, -8.9403) (-5.912, -8.5698) (-7.0389, -8.1452) (-7.6178, -8.1452) knots 0 0 0 1 2 2 2
  spline S216 degree 2 poles (-7.6178, -8.1452) (-8.2122, -8.1452) (-9.0304, -8.6469) (-9.0304, -9.1487) knots 0 0 0 1 2 2 2
  spline S217 degree 2 poles (-9.0304, -9.1487) (-9.0304, -9.6041) (-8.5441, -10.044) (-8.0038, -10.183) knots 0 0 0 1 2 2 2
  spline S218 degree 2 poles (-8.0038, -10.183) (-7.7413, -10.2524) (-7.0775, -10.3914) (-6.7147, -10.4763) knots 0 0 0 1 2 2 2
  spline S219 degree 2 poles (-6.7147, -10.4763) (-5.9274, -10.677) (-5.1247, -11.5955) (-5.1247, -12.3906) knots 0 0 0 1 2 2 2
  spline S220 degree 2 poles (-5.1247, -12.3906) (-5.1247, -12.8537) (-5.4874, -13.6719) (-5.8425, -13.9729) knots 0 0 0 1 2 2 2
  spline S221 degree 2 poles (-5.8425, -13.9729) (-6.2207, -14.2894) (-7.1856, -14.6213) (-7.9189, -14.6213) knots 0 0 0 1 2 2 2
  line L151 (-2.7781, -14.4515) -> (-3.9823, -14.4515)
  line L152 (-3.9823, -14.4515) -> (-3.9823, -7.3039)
  line L153 (-3.9823, -7.3039) -> (-2.7781, -7.3039)
  line L154 (-2.7781, -7.3039) -> (-2.7781, -14.4515)
  line L155 (-2.6932, -6.1152) -> (-4.0595, -6.1152)
  line L156 (-4.0595, -6.1152) -> (-4.0595, -4.8647)
  line L157 (-4.0595, -4.8647) -> (-2.6932, -4.8647)
  line L158 (-2.6932, -4.8647) -> (-2.6932, -6.1152)
  spline S222 degree 2 poles (4.8635, -10.8777) (4.8635, -12.6839) (3.1267, -14.6522) (1.6756, -14.6522) knots 0 0 0 1 2 2 2
  spline S223 degree 2 poles (1.6756, -14.6522) (0.1859, -14.6522) (-1.52, -12.6221) (-1.52, -10.8777) knots 0 0 0 1 2 2 2
  spline S224 degree 2 poles (-1.52, -10.8777) (-1.52, -9.0869) (0.2399, -7.1032) (1.6756, -7.1032) knots 0 0 0 1 2 2 2
  spline S225 degree 2 poles (1.6756, -7.1032) (3.1267, -7.1032) (4.8635, -9.0792) (4.8635, -10.8777) knots 0 0 0 1 2 2 2
  spline S226 degree 2 poles (3.6207, -10.8777) (3.6207, -9.4883) (2.6096, -8.1375) (1.6756, -8.1375) knots 0 0 0 1 2 2 2
  spline S227 degree 2 poles (1.6756, -8.1375) (0.7416, -8.1375) (-0.2773, -9.4883) (-0.2773, -10.8777) knots 0 0 0 1 2 2 2
  spline S228 degree 2 poles (-0.2773, -10.8777) (-0.2773, -12.2285) (0.7416, -13.6178) (1.6756, -13.6178) knots 0 0 0 1 2 2 2
  spline S229 degree 2 poles (1.6756, -13.6178) (2.6019, -13.6178) (3.6207, -12.2516) (3.6207, -10.8777) knots 0 0 0 1 2 2 2
  line L159 (11.71, -14.4515) -> (10.5059, -14.4515)
  line L160 (10.5059, -14.4515) -> (10.5059, -10.376)
  spline S230 degree 2 poles (10.5059, -10.376) (10.5059, -9.8819) (10.4133, -9.0329) (10.2743, -8.7782) knots 0 0 0 1 2 2 2
  spline S231 degree 2 poles (10.2743, -8.7782) (10.1277, -8.508) (9.6028, -8.2456) (9.1551, -8.2456) knots 0 0 0 1 2 2 2
  spline S232 degree 2 poles (9.1551, -8.2456) (8.7074, -8.2456) (7.758, -8.7241) (7.3026, -9.1101) knots 0 0 0 1 2 2 2
  line L161 (7.3026, -9.1101) -> (7.3026, -14.4515)
  line L162 (7.3026, -14.4515) -> (6.0985, -14.4515)
  line L163 (6.0985, -14.4515) -> (6.0985, -7.3039)
  line L164 (6.0985, -7.3039) -> (7.3026, -7.3039)
  line L165 (7.3026, -7.3039) -> (7.3026, -8.0989)
  spline S233 degree 2 poles (7.3026, -8.0989) (7.8429, -7.6126) (8.885, -7.1032) (9.4716, -7.1032) knots 0 0 0 1 2 2 2
  spline S234 degree 2 poles (9.4716, -7.1032) (10.5213, -7.1032) (11.71, -8.4926) (11.71, -9.8125) knots 0 0 0 1 2 2 2
  line L166 (11.71, -9.8125) -> (11.71, -14.4515)
  spline S235 degree 2 poles (23.2419, -9.689) (23.2419, -12.2516) (21.7522, -14.6522) (20.2007, -14.6522) knots 0 0 0 1 2 2 2
  spline S236 degree 2 poles (20.2007, -14.6522) (18.6261, -14.6522) (17.1518, -12.2053) (17.1518, -9.6967) knots 0 0 0 1 2 2 2
  spline S237 degree 2 poles (17.1518, -9.6967) (17.1518, -7.1186) (18.6415, -4.7335) (20.2007, -4.7335) knots 0 0 0 1 2 2 2
  spline S238 degree 2 poles (20.2007, -4.7335) (21.7676, -4.7335) (23.2419, -7.2035) (23.2419, -9.689) knots 0 0 0 1 2 2 2
  spline S239 degree 2 poles (21.6055, -12.5912) (21.7908, -12.1204) (21.9452, -10.6693) (21.9452, -9.689) knots 0 0 0 1 2 2 2
  spline S240 degree 2 poles (21.9452, -9.689) (21.9452, -8.7087) (21.7908, -7.2653) (21.5978, -6.779) knots 0 0 0 1 2 2 2
  spline S241 degree 2 poles (21.5978, -6.779) (21.4049, -6.2927) (20.7333, -5.791) (20.2007, -5.791) knots 0 0 0 1 2 2 2
  spline S242 degree 2 poles (20.2007, -5.791) (19.6681, -5.791) (18.9812, -6.2927) (18.7805, -6.7944) knots 0 0 0 1 2 2 2
  spline S243 degree 2 poles (18.7805, -6.7944) (18.5875, -7.2807) (18.4486, -8.7627) (18.4486, -9.6967) knots 0 0 0 1 2 2 2
  spline S244 degree 2 poles (18.4486, -9.6967) (18.4486, -10.7001) (18.5721, -12.0432) (18.7727, -12.5681) knots 0 0 0 1 2 2 2
  spline S245 degree 2 poles (18.7727, -12.5681) (18.958, -13.0621) (19.645, -13.5947) (20.2007, -13.5947) knots 0 0 0 1 2 2 2
  spline S246 degree 2 poles (20.2007, -13.5947) (20.7256, -13.5947) (21.4126, -13.093) (21.6055, -12.5912) knots 0 0 0 1 2 2 2
  line L167 (29.8569, -14.4515) -> (25.2102, -14.4515)
  line L168 (25.2102, -14.4515) -> (25.2102, -13.4789)
  line L169 (25.2102, -13.4789) -> (26.9392, -13.4789)
  line L170 (26.9392, -13.4789) -> (26.9392, -7.0955)
  line L171 (26.9392, -7.0955) -> (25.2102, -7.0955)
  line L172 (25.2102, -7.0955) -> (25.2102, -6.2232)
  spline S247 degree 2 poles (25.2102, -6.2232) (26.1905, -6.2232) (27.1168, -5.6675) (27.1785, -4.8956) knots 0 0 0 1 2 2 2
  line L173 (27.1785, -4.8956) -> (28.1665, -4.8956)
  line L174 (28.1665, -4.8956) -> (28.1665, -13.4789)
  line L175 (28.1665, -13.4789) -> (29.8569, -13.4789)
  line L176 (29.8569, -13.4789) -> (29.8569, -14.4515)
  constraints: 2 end point, 2 horizontal, 1 horizontal alignment, 1 other
extrude "Extrusion3" cut sketch "Sketch2" against normal blind 1.27
ref_plane "Work Plane1" through (19.05, 0, 0) normal (1, 0, 0) x (0, 1, 0)
ref_plane "Work Plane2" through (-19.05, 0, 0) normal (1, 0, 0) x (0, 1, 0)
split "Split1" plane through (-19.05, 0, 0) removes the side toward (-1, 0, 0)
split "Split2" plane through (19.05, 0, 0) removes the side toward (1, 0, 0)
equation "\"d0\" = insideDiameter"
equation "\"d1\" = wallThickness"
equation "\"d2\" = topThickness"
equation "\"d4\" = supportThickness"
equation "\"d6\" = textDepth"
equation "\"insideDiameter\" = 168.275"
equation "\"wallThickness\" = 4.7625"
equation "\"topThickness\" = 4.7625"
equation "\"supportThickness\" = 25.4"
equation "\"textDepth\" = 1.27"
body "Solid1"
